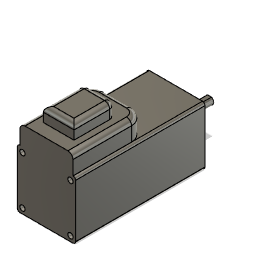
Assembly v15 (Autodesk Fusion 360 archive; units mm, degrees)
design "NEMA 23 Integrated Easy Servo Motor 130w"
Autodesk Fusion 360 part; units mm, degrees
sketch "Sketch1" plane through (0, 0, 0) normal (0, 0, 1) x (1, 0, 0)
  line L0 (0, 0) -> (57.15, 0)
  line L1 (57.15, 0) -> (57.15, 57.15)
  line L2 (57.15, 57.15) -> (0, 57.15)
  line L3 (0, 57.15) -> (0, 0)
  circle A0 centre (52.125, 52.125) radius 2.6
  line L4 (28.575, 0) -> (28.575, 57.15) construction
  line L5 (0, 28.575) -> (57.15, 28.575) construction
  circle A1 centre (5.025, 52.125) radius 2.6
  circle A2 centre (5.025, 5.025) radius 2.6
  circle A3 centre (52.125, 5.025) radius 2.6
  circle A4 centre (28.575, 28.575) radius 19.05
  line L6 (2.575, 57.15) -> (54.575, 57.15)
  line L7 (54.575, 57.15) -> (54.575, 76)
  line L8 (54.575, 76) -> (2.575, 76)
  line L9 (2.575, 76) -> (2.575, 57.15)
  circle A5 centre (28.575, 28.575) radius 4
  line L10 (26.6385, 32.075) -> (30.5115, 32.075)
  line L11 (13.575, 76) -> (43.575, 76)
  line L12 (43.575, 76) -> (43.575, 89.67)
  line L13 (43.575, 89.67) -> (13.575, 89.67)
  line L14 (13.575, 89.67) -> (13.575, 76)
  point P0 (47.5479, 45.3005)
  dimension "d1" = 57.15
  dimension "d2" = 57.15
  dimension "d3" = 5.2
  dimension "d5" = 5.2
  dimension "d6" = 47.1
  dimension "d8" = 5.2
  dimension "d10" = 47.1
  dimension "d12" = 5.2
  dimension "d13" = 47.1
  dimension "d14" = 47.1
  dimension "d15" = 38.1
  dimension "d16" = 76
  dimension "d17" = 8
  dimension "d19" = 3.5
  dimension "d20" = 52
  dimension "d21" = 13.67
  dimension "d22" = 30
  constraint horizontal L0
  constraint vertical L1
  constraint horizontal L2
  constraint vertical L3
  constraint coincident L0.start L3.end
  constraint midpoint L0 L4.start
  constraint midpoint L2 L4.end
  constraint midpoint L3 L5.start
  constraint midpoint L1 L5.end
  constraint symmetric A0 L4 A1
  constraint symmetric L5 A1.centre A2.centre
  constraint midpoint L5 A4.centre
  constraint horizontal L6
  constraint vertical L7
  constraint horizontal L8
  constraint vertical L9
  constraint coincident L2 L6.start
  constraint concentric A4 A5
  constraint coincident A5 L10.start
  constraint coincident A5 L10.end
  constraint perpendicular L4 L10
  constraint symmetric L4 L7 L9
  constraint horizontal L11
  constraint vertical L12
  constraint horizontal L13
  constraint vertical L14
  constraint coincident L8 L11.start
  constraint symmetric L4 L12 L14
  measures "d1" distance of L0.start L0.end
  measures "d2" distance of L0.start L2.end
  measures "d3" diameter of A0
  measures "d5" diameter of A1
  measures "d6" distance of A0.centre A1.centre
  measures "d8" diameter of A2
  measures "d10" distance of A1.centre A2.centre
  measures "d12" diameter of A3
  measures "d13" horizontal distance of A2.centre A3.centre
  measures "d14" distance of A0.centre A3.centre
  measures "d15" diameter of A4
  measures "d16" distance of L0 L8
  measures "d17" diameter of A5
  measures "d19" distance of L5 L10
  measures "d20" distance of L7.end L8.end
  measures "d21" distance of L11.start L13.end
  measures "d22" distance of L12.end L13.end
extrude "Extrude1" add sketch "Sketch1" along normal blind 127 contours L0 L1 L2 L3 L6 | A4 | A5 L10 | A5 L10
fillet "Fillet1" radius 2.5 4 edges at (57.15, 57.15, 63.5) (57.15, 0, 63.5) (0, 0, 63.5) (0, 57.15, 63.5)
extrude "Extrude2" add sketch "Sketch1" against normal blind 70 from surface at 127 contours L2 L6 L7 L8 L9 L11
fillet "Fillet2" radius 12.5 2 edges at (54.575, 66.575, 57) (2.575, 66.575, 57)
fillet "Fillet2" radius 5 3 edges at (54.575, 76, 92) (28.575, 76, 57) (2.575, 76, 92)
extrude "Extrude3" add sketch "Sketch1" along normal blind 40 from surface at 75 contours L8 L11 L12 L13 L14
fillet "Fillet3" radius 5 6 edges at (43.575, 89.67, 95) (43.575, 82.835, 75) (13.575, 82.835, 75) (28.575, 89.67, 75) (13.575, 89.67, 95) (28.575, 89.67, 115)
extrude "Extrude4" add sketch "Sketch1" against normal blind 2 contours A4 | A5 L10 | A5 L10
extrude "Extrude5" add sketch "Sketch1" against normal blind 33 contours A5 L10 picked at (29.5161, 29.5962)
extrude "Extrude6" add sketch "Sketch1" against normal blind 6 contours A5 L10 picked at (28.1041, 32.1557)
equation "d10 = d6"
equation "d12 = d3"
equation "d13 = d6"
equation "d14 = d6"
equation "d19 = 7.5 mm - ( d17 / 2 )"
equation "d44 = ( -1 * ( 33 - 27 ) ) * 1 mm"

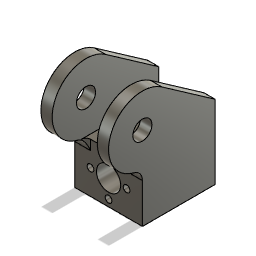
design "Lead Screw Nut Mount"
Autodesk Fusion 360 part; units mm, degrees
sketch "Sketch1" plane through (0, 0, 0) normal (0, 0, 1) x (1, 0, 0)
  circle A0 centre (0, 0) radius 5.375
  line L0 (0, 0) -> (0, 45)
  line L1 (0, 0) -> (55, 0)
  line L2 (-15, -11) -> (15, -11)
  line L3 (15, -11) -> (15, 11)
  line L4 (15, 11) -> (-15, 11)
  line L5 (-15, 11) -> (-15, -11)
  circle A1 centre (0, 8) radius 1.5
  circle A2 centre (-8, 0) radius 1.5
  circle A3 centre (0, -8) radius 1.5
  circle A4 centre (8, 0) radius 1.5
  dimension "d5" = 10.75
  dimension "d9" = 3
  dimension "d10" = 8
  dimension "d12" = 360
  dimension "d14" = 3
  dimension "d27" = 30
  constraint coincident A0.centre L0.start
  constraint vertical L0
  constraint perpendicular L0 L1
  constraint horizontal L2
  constraint vertical L3
  constraint horizontal L4
  constraint vertical L5
  constraint symmetric L0 L3 L5
  constraint symmetric L1 L2 L4
  constraint coincident L0 A1.centre
  measures "d5" diameter of A0
  measures "d9" diameter of A1
  measures "d10" distance of A0.centre A1.centre
  measures "d14" distance of L2 A3.centre
  measures "d27" distance of L3 L5
extrude "Extrude1" add sketch "Sketch1" along normal blind 32.25 contours A0 L0 L1 L2 L3 L4 L5 A1 A4 | A0 L0 L1 L3 L4 A1 A4
sketch "Sketch2" plane through (15, 0, 0) normal (1, 0, 0) x (0, 0, -1)
  line L0 (0, -11) -> (0, 11)
  line L1 (0, 11) -> (-32.25, 11)
  line L2 (-32.25, 11) -> (-32.25, -11)
  line L3 (-32.25, -11) -> (0, -11)
  circle A0 centre (-32.25, 26) radius 4.25
  circle A1 centre (-32.25, 26) radius 15
  line L4 (0, 11) -> (0, 21.7299)
  line L5 (0, 21.7299) -> (-23.6464, 38.2873)
  dimension "d20" = 8.5
  dimension "d21" = 15
  dimension "d28" = 30
  dimension "d34" = 125
  constraint concentric A0 A1
  constraint coincident L1.end A1
  constraint coincident L0.end L1.start
  constraint perpendicular L1 L4
  constraint coincident A1 L5.end
  constraint tangent A1 L5
  measures "d20" diameter of A0
  measures "d21" distance of L1 A0.centre
  measures "d28" diameter of A1
  measures "d34" angle of L4 L5
extrude "Extrude2" add sketch "Sketch2" against normal blind 5 contours L1 A1 L4 L5 | A1
ref_plane "WorkPlane1" through (0, 16.75, 24.9478) normal (1, 0, 0) x (0, 1, 0)
mirror "Mirror1" about plane through (0, 16.75, 24.9478) normal (1, 0, 0) of "Extrude2"
fillet "Fillet1" radius 5 2 edges at (-12.5, 11, 32.25) (12.5, 11, 32.25)
fillet "Fillet2" radius 2 1 edges at (-10, 8.8175, 32.25)
equation "Screw_Nut_Dia = 10 mm"
equation "Screw_Nut_bolt_Dia = 3 mm"
equation "Screw_Nut_Bolt_Pattern = 16 mm"
equation "d5 = Screw_Nut_Dia + 0.75 mm"
equation "d9 = Screw_Nut_bolt_Dia"
equation "d10 = Screw_Nut_Bolt_Pattern / 2"
equation "d13 = Screw_Nut_bolt_Dia"
equation "d14 = d13"
equation "d28 = 22 mm + 8 mm"
equation "d34 = 180 deg - 55 deg"

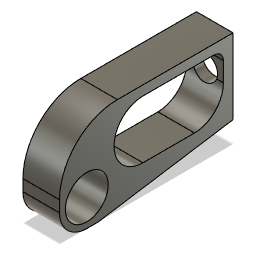
design "Connector 2"
Autodesk Fusion 360 part; units mm, degrees
sketch "Sketch1" plane through (0, 0, 0) normal (0, 1, 0) x (1, 0, 0)
  line L0 (0, 0) -> (19, 0)
  line L1 (19, 0) -> (19, 90)
  line L2 (19, 90) -> (0, 90)
  line L3 (0, 90) -> (0, 0)
  dimension "d1" = 19
  dimension "d2" = 90
  constraint horizontal L0
  constraint vertical L1
  constraint horizontal L2
  constraint vertical L3
  constraint coincident L0.start L3.end
  measures "d1" distance of L0.start L0.end
  measures "d2" distance of L0.start L2.end
extrude "Extrude1" add sketch "Sketch1" along normal blind 50
sketch "Sketch2" plane through (19, 0, 0) normal (1, 0, 0) x (0, 0, -1)
  line L0 (0, 0) -> (90, 0)
  line L1 (90, 0) -> (90, 50)
  line L2 (90, 50) -> (0, 50)
  line L3 (0, 50) -> (0, 0)
  circle A0 centre (14.125, 14.125) radius 11.125
  line L4 (28.25, 45) -> (85, 45)
  line L5 (85, 45) -> (85, 15)
  line L6 (85, 15) -> (28.25, 15)
  line L7 (28.25, 15) -> (28.25, 45)
  circle A1 centre (14.125, 14.125) radius 14.125
  dimension "d5" = 22.25
  dimension "d7" = 5
  dimension "d8" = 15
  dimension "d9" = 5
  dimension "d10" = 30
  dimension "d24" = 3
  constraint horizontal L4
  constraint vertical L5
  constraint horizontal L6
  constraint vertical L7
  constraint tangent L3 A1
  constraint tangent L0 A1
  constraint tangent L7 A1
  measures "d5" diameter of A0
  measures "d7" distance of L2 L4
  measures "d8" distance of L0 L6
  measures "d9" distance of L1 L5
  measures "d10" distance of L4 L6
extrude "Extrude2" cut sketch "Sketch2" against normal up to surface (19 mm away) contours L0 L3 A1 | A0 | L4 L5 L6 L7
fillet "Fillet1" radius 30 1 edges at (9.5, 50, 0)
sketch "Sketch3" plane through (0, 0, -90) normal (0, 0, -1) x (-1, 0, 0)
  line L0 (-19, 0) -> (0, 0)
  line L1 (0, 0) -> (0, 50)
  line L2 (0, 50) -> (-19, 50)
  line L3 (-19, 50) -> (-19, 0)
  circle A0 centre (-9.5, 32.5) radius 6.5
  line L4 (-9.5, 50) -> (-9.5, 0) construction
  line L5 (-19, 32.5) -> (0, 32.5) construction
  dimension "d17" = 13
  dimension "d29" = 17.5
  constraint midpoint L2 L4.start
  constraint midpoint L0 L4.end
  constraint coincident A0.centre L4
  constraint coincident A0.centre L5
  constraint horizontal L5
  constraint coincident L3 L5.start
  constraint coincident L1 L5.end
  measures "d17" diameter of A0
  measures "d29" distance of L2 L5
extrude "Extrude3" cut sketch "Sketch3" against normal up to surface (5 mm away) contours A0
fillet "Fillet2" radius 15 1 edges at (9.5, 15, -85)
fillet "Fillet2" radius 5 1 edges at (9.5, 45, -85)
fillet "Fillet3" radius 15 2 edges at (9.5, 45, -28.25) (9.5, 15, -28.25)
chamfer "Chamfer1" distance 11 distance2 70 1 edges at (9.5, 0, -90) measured on face at (9.6619, 8.6727, -90)
equation "d6 = d5"

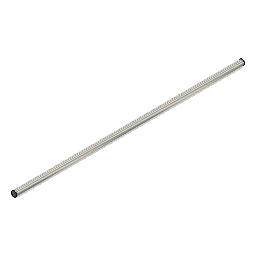
design "8mm T8 Lead Screw (345mm)"
Autodesk Fusion 360 part; units mm, degrees
sketch "Sketch1" plane through (0, 0, 0) normal (0, 0, 1) x (1, 0, 0)
  circle A0 centre (0, 0) radius 4
  dimension "d1" = 8
  constraint coincident A0.centre origin
  measures "d1" diameter of A0
extrude "Extrude1" add sketch "Sketch1" along normal blind 345
thread "Thread1" "ISO Metric Trapezoidal Threads 8.0 TR8x1.5 7e" major diameter 7.925 minor diameter 6.0605 pitch 1.5 angle 30 resizes the face on face at (-1.5959, -3.6679, 230)

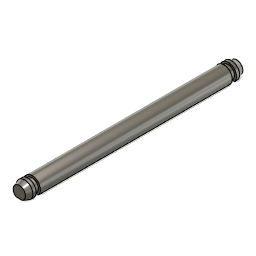
design "Pin Long (80mm)"
Autodesk Fusion 360 part; units mm, degrees
sketch "Sketch1" plane through (0, 0, 0) normal (0, 0, 1) x (1, 0, 0)
  line L0 (0, 0) -> (5.9867, 0)
  arc A0 (5.9867, 0) -> (0, 0) centre (2.9933, 2.5) ccw
  arc A1 (4.6516, 0) -> (1.335, 0) centre (2.9933, 2.5) ccw
  arc A2 (17.1516, 0) -> (13.835, 0) centre (15.4933, 2.5) ccw
  line L1 (12.5, 0) -> (18.4867, 0)
  arc A3 (18.4867, 0) -> (12.5, 0) centre (15.4933, 2.5) ccw
  arc A4 (29.6516, 0) -> (26.335, 0) centre (27.9933, 2.5) ccw
  line L2 (25, 0) -> (30.9867, 0)
  arc A5 (30.9867, 0) -> (25, 0) centre (27.9933, 2.5) ccw
  point P0 (12.5, 0)
  point P1 (25, 0)
  dimension "d1" = 3.9
  dimension "d2" = 2.5
  dimension "d13" = 6
  dimension "d16" = 25
  dimension "d17" = 0
  constraint coincident L0.start A0.end
  constraint horizontal L0
  constraint concentric A0 A1
  constraint coincident L0 A1.end
  constraint coincident L0 A1.start
  measures "d1" radius of A0
  measures "d2" distance of L0 A0.centre
  measures "d13" diameter of A1
extrude "Extrude1" add sketch "Sketch1" along normal blind 102 contours L0 A0 A1 | L0 A1 makes body 1
extrude "Extrude2" cut sketch "Sketch1" against normal blind 2 from surface at 6 contours L0 A0 A1 bodies 1
ref_plane "WorkPlane1" through (2.9933, 3.9289, 51) normal (0, 0, 1) x (1, 0, 0)
mirror "Mirror1" about plane through (2.9933, 3.9289, 51) normal (0, 0, 1) of "Extrude2"
extrude "Extrude3" add sketch "Sketch1" along normal blind 41 separate body contours A2 L1 | A2 L1 A3 makes body 2
extrude "Extrude4" cut sketch "Sketch1" against normal blind 2 from surface at 6 contours A2 L1 A3 bodies 2
ref_plane "WorkPlane2" through (15.4933, 3.9289, 20.5) normal (0, 0, 1) x (1, 0, 0)
mirror "Mirror2" about plane through (15.4933, 3.9289, 20.5) normal (0, 0, 1) of "Extrude4"
chamfer "Chamfer3" distance 2.5 distance2 1 1 edges at (15.4933, 6.4, 0) measured on face at (12.3817, 0.1488, 2.6667) on bodies 1 2
chamfer "Chamfer3" distance 2.5 distance2 1 1 edges at (2.9933, 6.4, 0) measured on face at (-0.1183, 0.1488, 2.6667) on bodies 1 2
chamfer "Chamfer3" distance 1 distance2 2.5 2 edges at (15.4933, 6.4, 41) (2.9933, 6.4, 102) measured on face at (16.772, 1.0681, 41) measured on face at (3.5688, 2.2017, 102) on bodies 1 2
hidden bodies 2
equation "d7 = Long_Pin + End_Thickness * 2"
equation "C_Clip_Thickness = 2 mm"
equation "End_Thickness = 4 mm + C_Clip_Thickness"
equation "Long_Pin = 90 mm"
equation "Short_Pin = 29 mm"
equation "d18 = End_Thickness"
equation "d19 = -C_Clip_Thickness"
equation "d25 = Short_Pin + End_Thickness * 2"
equation "d27 = End_Thickness"
equation "d28 = -C_Clip_Thickness"

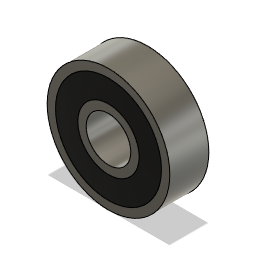
design "608 Bearings"
Autodesk Fusion 360 part; units mm, degrees
sketch "Sketch1" plane through (0, 0, 0) normal (0, 0, 1) x (1, 0, 0)
  circle A0 centre (0, 0) radius 11
  circle A1 centre (0, 0) radius 9.5
  circle A2 centre (0, 0) radius 4
  circle A3 centre (0, 0) radius 5.5
  dimension "d1" = 22
  dimension "d2" = -1.5
  dimension "d3" = 8
  dimension "d4" = 1.5
  constraint coincident A0.centre A1.centre
  measures "d1" diameter of A0
  measures "d3" diameter of A2
extrude "Extrude1" add sketch "Sketch1" along normal blind 7 makes body 1 at (5.4727, -0.5476, 4.6667) makes body 2 at (10.9453, -1.0952, 4.6667)
extrude "Extrude2" add sketch "Sketch1" along normal blind 7 separate body contours A1 makes body 3

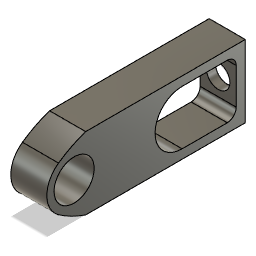
design "Connectors"
Autodesk Fusion 360 part; units mm, degrees
sketch "Sketch1" plane through (0, 0, 0) normal (0, 1, 0) x (1, 0, 0)
  line L0 (0, 0) -> (20, 0)
  line L1 (20, 0) -> (20, 110)
  line L2 (20, 110) -> (0, 110)
  line L3 (0, 110) -> (0, 0)
  dimension "d1" = 20
  dimension "d2" = 110
  constraint horizontal L0
  constraint vertical L1
  constraint horizontal L2
  constraint vertical L3
  constraint coincident L0.start L3.end
  measures "d1" distance of L0.start L0.end
  measures "d2" distance of L0.start L2.end
extrude "Extrude1" add sketch "Sketch1" along normal blind 40
sketch "Sketch2" plane through (20, 0, 0) normal (1, 0, 0) x (0, 0, -1)
  line L0 (0, 0) -> (110, 0)
  line L1 (110, 0) -> (110, 40)
  line L2 (110, 40) -> (0, 40)
  line L3 (0, 40) -> (0, 0)
  circle A0 centre (15.125, 20) radius 11.125
  line L4 (60, 35) -> (105, 35)
  line L5 (105, 35) -> (105, 5)
  line L6 (105, 5) -> (60, 5)
  line L7 (60, 5) -> (60, 35)
  line L8 (0, 20) -> (13, 20) construction
  circle A1 centre (15.125, 20) radius 15.125
  arc A2 (60, 40) -> (6.4846, 32.414) centre (40.7607, -16.8318) ccw
  arc A3 (6.4846, 7.586) -> (60, 0) centre (40.7607, 56.8318) ccw
  dimension "d5" = 22.25
  dimension "d7" = 5
  dimension "d8" = 5
  dimension "d9" = 5
  dimension "d10" = 30
  dimension "d11" = 45
  dimension "d24" = 4
  dimension "d25" = 60
  constraint horizontal L4
  constraint vertical L5
  constraint horizontal L6
  constraint vertical L7
  constraint midpoint L3 L8.start
  constraint perpendicular L3 L8
  constraint coincident A0.centre L8
  constraint tangent A1 A2
  constraint coincident A1 A2.end
  constraint coincident L2 A2.start
  constraint coincident L7 A2.start
  constraint symmetric L8 A2.start A3.end
  constraint symmetric L8 A2.end A3.start
  constraint symmetric L8 A2 A3
  constraint tangent L3 A1
  measures "d5" diameter of A0
  measures "d7" distance of L2 L4
  measures "d8" distance of L0 L6
  measures "d9" distance of L1 L5
  measures "d10" distance of L4 L6
  measures "d11" distance of L5 L7
  measures "d25" radius of A2
extrude "Extrude2" cut sketch "Sketch2" against normal up to surface (20 mm away) contours L0 L3 A1 A3 | L2 L3 A1 A2 | A0 | L4 L5 L6 L7
sketch "Sketch3" plane through (0, 0, -110) normal (0, 0, -1) x (-1, 0, 0)
  line L0 (-20, 0) -> (0, 0)
  line L1 (0, 0) -> (0, 40)
  line L2 (0, 40) -> (-20, 40)
  line L3 (-20, 40) -> (-20, 0)
  circle A0 centre (-10, 20) radius 6.5
  line L4 (-10, 40) -> (-10, 0) construction
  line L5 (-20, 20) -> (0, 20) construction
  dimension "d17" = 13
  constraint midpoint L2 L4.start
  constraint midpoint L0 L4.end
  constraint midpoint L3 L5.start
  constraint midpoint L1 L5.end
  constraint coincident A0.centre L4
  constraint coincident A0.centre L5
  measures "d17" diameter of A0
extrude "Extrude3" cut sketch "Sketch3" against normal up to surface (5 mm away) contours A0
fillet "Fillet2" radius 5 2 edges at (10, 35, -105) (10, 5, -105)
fillet "Fillet3" radius 15 2 edges at (10, 35, -60) (10, 5, -60)

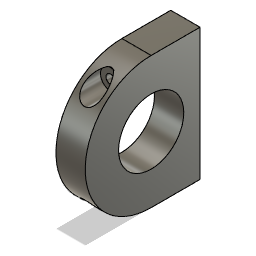
design "Pedal Mounting Ears"
Autodesk Fusion 360 part; units mm, degrees
sketch "Sketch1" plane through (0, 0, 0) normal (1, 0, 0) x (0, 0, -1)
  line L0 (-16.6875, 45) -> (0, 45)
  line L1 (0, 45) -> (0, 0)
  line L2 (0, 0) -> (-16.6875, 0)
  arc A0 (-16.6875, 45) -> (-16.6875, 0) centre (-16.6875, 22.5) ccw
  circle A1 centre (-16.6875, 22.5) radius 11.125
  line L3 (0, 22.5) -> (-29, 22.5) construction
  circle A2 centre (-16.6875, 22.5) radius 9.125
  dimension "d1" = 22.25
  dimension "d2" = 45
  dimension "d3" = 16.6875
  dimension "d4" = -2
  constraint horizontal L0
  constraint coincident L1.end L2.start
  constraint perpendicular L0 L1
  constraint perpendicular L1 L2
  constraint tangent L2 A0
  constraint tangent L0 A0
  constraint midpoint L1 L3.start
  constraint perpendicular L1 L3
  constraint coincident A0.centre L3
  constraint coincident A0.centre A1.centre
  measures "d1" diameter of A1
  measures "d2" distance of L0 L2
  measures "d3" distance of L1 A0.centre
extrude "Extrude2" add sketch "Sketch1" along normal blind 10 contours L0 L1 L2 A0
sketch "Sketch2" plane through (0, 0, 0) normal (0, 0, -1) x (-1, 0, 0)
  line L0 (0, 45) -> (-10, 45)
  line L1 (-10, 0) -> (0, 0)
  circle A0 centre (-5, 5.2) radius 3.5
  line L2 (-5, 0) -> (-5, 4) construction
  circle A1 centre (-5, 5.2) radius 1.6
  line L3 (0, 0) -> (0, 45)
  line L4 (-10, 45) -> (-10, 0)
  dimension "d13" = 7
  dimension "d14" = 5.2
  dimension "d17" = 3.2
  constraint midpoint L1 L2.start
  constraint perpendicular L1 L2
  constraint coincident A0.centre L2
  constraint concentric A0 A1
  measures "d13" diameter of A0
  measures "d14" distance of L1 A0.centre
  measures "d17" diameter of A1
extrude "Extrude4" cut sketch "Sketch2" against normal blind 40 contours A0 | A1
extrude "Extrude5" add sketch "Sketch2" against normal blind 25.5 contours A0
ref_plane "WorkPlane1" through (5, 22.5, 8.3438) normal (0, -1, 0) x (0, 0, -1)
mirror "Mirror1" about plane through (5, 22.5, 8.3438) normal (0, -1, 0) of "Extrude4", "Extrude5"
equation "d3 = d1 * 0.75"
equation "d14 = d13 / 2 + 1.7 mm"

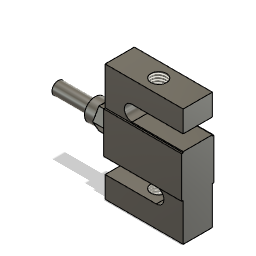
design "Load Cell (300 kg)"
Autodesk Fusion 360 part; units mm, degrees
sketch "Sketch1" plane through (0, 0, 0) normal (0, 0, 1) x (1, 0, 0)
  line L0 (0, 0) -> (50.75, 0)
  line L1 (50.75, 0) -> (50.75, 52.25)
  line L2 (50.75, 52.25) -> (12.5, 52.25)
  line L3 (12.5, 52.25) -> (12.5, 62.25)
  line L4 (12.5, 62.25) -> (50.75, 62.25)
  line L5 (50.75, 62.25) -> (50.75, 76.25)
  line L6 (50.75, 76.25) -> (0, 76.25)
  line L7 (0, 76.25) -> (0, 24)
  line L8 (0, 24) -> (38.25, 24)
  line L9 (38.25, 24) -> (38.25, 14)
  line L10 (38.25, 14) -> (0, 14)
  line L11 (0, 14) -> (0, 0)
  line L12 (0, 24.75) -> (50.75, 24.75)
  line L13 (50.75, 51.5) -> (0, 51.5)
  dimension "d1" = 76.25
  dimension "d2" = 14
  dimension "d3" = 10
  dimension "d4" = 50.75
  dimension "d5" = 12.5
  dimension "d6" = 0.75
  dimension "d7" = 0.75
  constraint coincident L0.start L11.end
  constraint horizontal L0
  constraint perpendicular L0 L1
  constraint perpendicular L1 L2
  constraint perpendicular L2 L3
  constraint perpendicular L3 L4
  constraint perpendicular L4 L5
  constraint perpendicular L5 L6
  constraint perpendicular L6 L7
  constraint perpendicular L7 L8
  constraint perpendicular L8 L9
  constraint perpendicular L9 L10
  constraint perpendicular L0 L11
  constraint equal L5 L11
  constraint equal L3 L9
  constraint collinear L7 L11
  constraint collinear L1 L5
  constraint equal L2 L10
  constraint coincident L7 L12.start
  constraint coincident L1 L12.end
  constraint perpendicular L1 L12
  constraint coincident L1 L13.start
  constraint coincident L7 L13.end
  constraint perpendicular L7 L13
  measures "d1" distance of L0 L6
  measures "d2" distance of L4.end L5.end
  measures "d3" distance of L2.end L3.end
  measures "d4" distance of L5.end L6.end
  measures "d5" distance of L1 L9
  measures "d6" distance of L8 L12
  measures "d7" distance of L2 L13
extrude "Extrude1" add sketch "Sketch1" along normal mid plane 19
extrude "Extrude2" add sketch "Sketch1" along normal mid plane 21 contours L1 L7 L12 L13
sketch "Sketch2" plane through (0, 0, 0) normal (-1, 0, 0) x (0, 0, 1)
  line L0 (9.5, 51.5) -> (9.5, 76.25)
  line L1 (9.5, 76.25) -> (-9.5, 76.25)
  line L2 (-9.5, 76.25) -> (-9.5, 51.5)
  line L3 (-9.5, 51.5) -> (-10.5, 51.5)
  line L4 (-10.5, 51.5) -> (-10.5, 24.75)
  line L5 (-10.5, 24.75) -> (-9.5, 24.75)
  line L6 (-9.5, 24.75) -> (-9.5, 24)
  line L7 (-9.5, 24) -> (9.5, 24)
  line L8 (9.5, 24) -> (9.5, 24.75)
  line L9 (9.5, 24.75) -> (10.5, 24.75)
  line L10 (10.5, 24.75) -> (10.5, 51.5)
  line L11 (10.5, 51.5) -> (9.5, 51.5)
  line L12 (8.0829, 38.125) -> (4.0415, 45.125)
  line L13 (4.0415, 45.125) -> (-4.0415, 45.125)
  line L14 (-4.0415, 45.125) -> (-8.0829, 38.125)
  line L15 (-8.0829, 38.125) -> (-4.0415, 31.125)
  line L16 (-4.0415, 31.125) -> (4.0415, 31.125)
  line L17 (4.0415, 31.125) -> (8.0829, 38.125)
  line L18 (-9.5, 0) -> (9.5, 0)
  line L19 (0, 76.25) -> (0, 24)
  circle A0 centre (0, 38.125) radius 4.1
  circle A1 centre (0, 38.125) radius 7
  point P0 (0, 38.125)
  dimension "d12" = 7
  dimension "d13" = 38.125
  dimension "d14" = 8.2
  dimension "d15" = 14
  constraint horizontal L16
  constraint coincident P0 L19
  constraint coincident P0 A0.centre
  constraint concentric A0 A1
  measures "d12" distance of P0 L17
  measures "d13" distance of P0 L18
  measures "d14" diameter of A0
  measures "d15" diameter of A1
extrude "Extrude3" add sketch "Sketch2" along normal blind 9.5 contours L13 L14 A1 | L19 A0 A1 | L12 L13 A1 | L19 A0 A1 | L19 A0 | L19 A0 | L12 L17 A1 | L14 L15 A1 | L15 L16 A1 | L16 L17 A1
extrude "Extrude4" add sketch "Sketch2" along normal blind 16 contours L19 A0 A1 | L19 A0 A1 | L19 A0 | L19 A0
extrude "Extrude5" add sketch "Sketch2" along normal blind 40 contours L19 A0 | L19 A0
fillet "Fillet1" radius 5 4 edges at (38.25, 14, 0) (38.25, 24, 0) (12.5, 62.25, 0) (12.5, 52.25, 0)
sketch "Sketch3" plane through (0, 76.25, 0) normal (0, 1, 0) x (-1, 0, 0)
  line L0 (0, -9.5) -> (0, 9.5)
  line L1 (0, 9.5) -> (-50.75, 9.5)
  line L2 (-50.75, 9.5) -> (-50.75, -9.5)
  line L3 (-50.75, -9.5) -> (0, -9.5)
  circle A0 centre (-25.375, 0) radius 6
  line L4 (0, 4.0415) -> (0, -4.0415)
  line L5 (-50.75, 0) -> (0, 0)
  dimension "d24" = 25.375
  dimension "d25" = 12
  constraint coincident A0.centre L5
  measures "d24" distance of A0.centre L4
  measures "d25" diameter of A0
extrude "Extrude6" cut sketch "Sketch3" against normal up to surface (14 mm away) contours A0 L5 | A0 L5
extrude "Extrude7" cut sketch "Sketch3" along normal up to surface (14 mm away) from surface at -76.25 contours A0 L5 | A0 L5
thread "Thread1" "ISO Metric profile 12.0 M12x1.75 6H" major diameter 12.2265 minor diameter 10.2735 pitch 1.75 angle 60 resizes the face on face at (19.3825, 66.9167, -0.2991)
thread "Thread2" "ISO Metric profile 12.0 M12x1.75 6H" major diameter 12.2265 minor diameter 10.2735 pitch 1.75 angle 60 resizes the face on face at (19.4048, 4.6667, -0.5974)
equation "d8 = ( 19 / 2 ) * 1 mm"
equation "d10 = ( 21 / 2 ) * 1 mm"
equation "d12 = ( 14 / 2 ) * 1 mm"
equation "d13 = d1 / 2"
equation "d24 = d4 / 2"

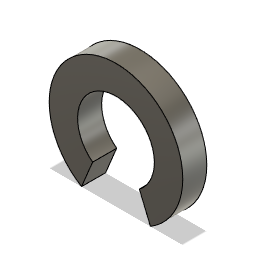
design "C Clip"
Autodesk Fusion 360 part; units mm, degrees
sketch "Sketch1" plane through (0, 0, 0) normal (0, 0, 1) x (1, 0, 0)
  line L0 (-1.75, -2.281) -> (-2.5794, -4.2833)
  line L1 (1.75, -2.281) -> (2.5794, -4.2833)
  line L2 (0, 0) -> (0, -5) construction
  arc A0 (2.5794, -4.2833) -> (-2.5794, -4.2833) centre (0, 0) ccw
  arc A1 (1.75, -2.281) -> (-1.75, -2.281) centre (0, 0) ccw
  dimension "d7" = 5.75
  dimension "d8" = 10
  dimension "d9" = 45
  dimension "d10" = 3.5
  constraint coincident L2.start A0.centre
  constraint concentric A0 A1
  constraint vertical L2
  constraint symmetric L0 L1 L2
  measures "d7" diameter of A1
  measures "d8" diameter of A0
  measures "d9" angle of L0 L1
  measures "d10" distance of L1.start L0.start
extrude "Extrude1" add sketch "Sketch1" along normal blind 1.8

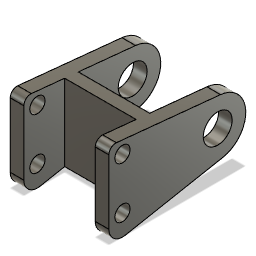
design "Pedal Connector"
Autodesk Fusion 360 part; units mm, degrees
sketch "Sketch3" plane through (0, 0, 0) normal (1, 0, 0) x (0, 0, -1)
  circle A0 centre (4, 22) radius 2.25
  circle A1 centre (4, 7) radius 2.25
  line L0 (0, 0) -> (0, 26)
  circle A2 centre (32, 14.5) radius 4.25
  line L1 (12, 24.7968) -> (12, 2.288)
  line L2 (4, 22) -> (4, 7) construction
  line L3 (4, 14.5) -> (32, 14.5) construction
  circle A3 centre (32, 14.5) radius 8.25
  line L4 (0, 26) -> (32.8231, 22.7088)
  line L5 (0, 0) -> (33.5452, 6.396)
  line L6 (16, 24.3957) -> (16, 0.2355)
  dimension "d16" = 4.5
  dimension "d17" = 4.5
  dimension "d18" = 8.5
  dimension "d21" = 4
  dimension "d22" = 4
  dimension "d23" = 15
  dimension "d25" = 4
  dimension "d28" = 8
  dimension "d29" = 7
  dimension "d30" = 90
  dimension "d32" = 4
  dimension "d43" = 4
  dimension "d44" = 16
  constraint coincident L0.start L5.start
  constraint vertical L0
  constraint coincident A0.centre L2.start
  constraint coincident A1.centre L2.end
  constraint midpoint L2 L3.start
  constraint coincident A2.centre L3.end
  constraint parallel L0 L1
  constraint coincident A3 L4.end
  constraint tangent A3 L4
  constraint coincident A3 L5.end
  constraint tangent A3 L5
  constraint coincident L1.start L4
  constraint coincident L1.end L5
  constraint coincident L4 L6.start
  constraint vertical L6
  measures "d16" diameter of A0
  measures "d17" diameter of A1
  measures "d18" diameter of A2
  measures "d21" distance of A1.centre L0
  measures "d22" distance of A0.centre L0
  measures "d23" distance of A0.centre A1.centre
  measures "d25" vertical distance of A0.centre L0.end
  measures "d28" distance of A0.centre L1
  measures "d29" vertical distance of L0.start A1.centre
  measures "d30" angle of L2 L3
  measures "d43" distance of L1 L6
  measures "d44" distance of A2.centre L6
extrude "Extrude2" add sketch "Sketch3" along normal blind 29
fillet "Fillet1" radius 4 1 edges at (14.5, 0, 0)
fillet "Fillet1" radius 2 1 edges at (14.5, 26, 0)
extrude "Extrude3" cut sketch "Sketch3" along normal blind 21 from surface at 4 contours L0 L1 L4 L5 | A3 L4 L5 L6 | A3
equation "d19 = d18 / 2 + 4 mm"
equation "d34 = 21 mm + ( 4 * 2 ) * 1 mm"
equation "d44 = ( 22 / 2 ) * 1 mm + 5 mm"

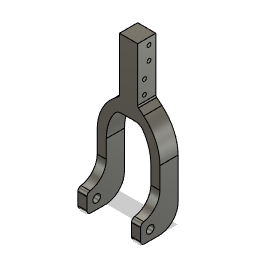
design "Pedal"
Autodesk Fusion 360 part; units mm, degrees
sketch "Pedal Shape" plane through (0, 0, 0) normal (0, 0, 1) x (1, 0, 0)
  line L0 (0, 0) -> (0, 89.4421)
  line L1 (0, 89.4421) -> (24.5, 110)
  line L2 (24.5, 110) -> (24.5, 170)
  line L3 (24.5, 170) -> (44.5, 170)
  line L4 (44.5, 170) -> (44.5, 110)
  line L5 (44.5, 110) -> (69, 89.4421)
  line L6 (69, 89.4421) -> (69, 0)
  line L7 (69, 0) -> (59, 0)
  line L8 (59, 0) -> (59, 84.779)
  line L9 (59, 84.779) -> (47.0825, 94.779)
  line L10 (47.0825, 94.779) -> (21.9175, 94.779)
  line L11 (21.9175, 94.779) -> (10, 84.779)
  line L12 (10, 84.779) -> (10, 0)
  line L13 (10, 0) -> (0, 0)
  dimension "d2" = 20
  dimension "d4" = 10
  dimension "d6" = 170
  dimension "d7" = 10
  dimension "d45" = 10
  dimension "d47" = 110
  dimension "d48" = 69
  constraint parallel L0 L2
  constraint perpendicular L2 L3
  constraint perpendicular L3 L4
  constraint perpendicular L3 L6
  constraint perpendicular L6 L7
  constraint perpendicular L7 L8
  constraint parallel L5 L9
  constraint perpendicular L8 L10
  constraint perpendicular L10 L12
  constraint coincident L0.start L13.end
  constraint equal L7 L13
  constraint equal L9 L11
  constraint equal L8 L12
  constraint equal L1 L5
  constraint equal L2 L4
  constraint horizontal L13
  constraint horizontal L7
  constraint collinear L7 L13
  constraint parallel L1 L11
  measures "d2" distance of L2.end L3.end
  measures "d4" distance of L0 L12
  measures "d6" distance of L3 L13
  measures "d7" distance of L5 L9
  measures "d45" distance of L10 L11.end
  measures "d47" distance of L1.end L13
  measures "d48" distance of L0 L6
extrude "Extrude1" add sketch "Pedal Shape" along normal blind 20
sketch "Pivot Point" plane through (0, 0, 0) normal (-1, 0, 0) x (0, 0, 1)
  line L0 (0, 89.4421) -> (0, 0)
  line L1 (0, 0) -> (20, 0)
  line L2 (20, 0) -> (20, 89.4421)
  line L3 (20, 89.4421) -> (0, 89.4421)
  circle A0 centre (30.625, 10.625) radius 4.25
  line L4 (20, 21.25) -> (41.25, 21.25)
  line L5 (41.25, 21.25) -> (41.25, 0)
  line L6 (41.25, 0) -> (20, 0)
  line L7 (20, 21.25) -> (20, 0)
  line L8 (30.625, 21.25) -> (30.625, 0) construction
  dimension "d12" = 8.5
  dimension "d13" = 10.625
  dimension "d16" = 21.25
  dimension "d17" = 21.25
  constraint coincident L2 L4.start
  constraint perpendicular L2 L4
  constraint perpendicular L4 L5
  constraint coincident L1.end L2.start
  constraint perpendicular L2 L6
  constraint midpoint L4 L8.start
  constraint midpoint L6 L8.end
  constraint coincident A0.centre L8
  measures "d12" diameter of A0
  measures "d13" distance of L1 A0.centre
  measures "d16" distance of L4.end L5.end
  measures "d17" distance of L5 L7
extrude "Extrude3" add sketch "Pivot Point" against normal blind 10 contours L2 L4 L5 L6 L7
fillet "Fillet1" radius 21.25 1 edges at (5, 21.25, 20)
fillet "Fillet1" radius 21.25 1 edges at (5, 0, 0)
ref_plane "WorkPlane1" through (34.5, 44.721, 10) normal (1, 0, 0) x (0, 1, 0)
mirror "Mirror1" about plane through (34.5, 44.721, 10) normal (1, 0, 0) of "Extrude3", "Fillet1"
sketch "Pedal and Connector Holes" plane through (44.5, 0, 0) normal (1, 0, 0) x (0, 0, -1)
  line L0 (0, 110) -> (0, 170)
  line L1 (0, 170) -> (-20, 170)
  line L2 (-20, 170) -> (-20, 110)
  line L3 (-20, 110) -> (0, 110)
  circle A0 centre (-12.5, 117.5) radius 2.125
  circle A1 centre (-12.5, 132.5) radius 2.125
  line L4 (-12.5, 105) -> (-12.5, 132.5) construction
  circle A2 centre (-7.5, 162.5) radius 2.125
  circle A3 centre (-7.5, 147.5) radius 2.125
  line L5 (-7.5, 162.5) -> (-7.5, 147.5) construction
  dimension "d27" = 4.25
  dimension "d28" = 4.25
  dimension "d29" = 15
  dimension "d30" = 7.5
  dimension "d33" = 7.5
  dimension "d34" = 4.25
  dimension "d35" = 4.25
  dimension "d36" = 15
  dimension "d37" = 7.5
  dimension "d38" = 7.5
  constraint coincident A1.centre L4.end
  constraint coincident A0.centre L4
  constraint vertical L4
  constraint coincident A2.centre L5.start
  constraint coincident A3.centre L5.end
  constraint vertical L5
  measures "d27" diameter of A0
  measures "d28" diameter of A1
  measures "d29" distance of A0.centre A1.centre
  measures "d30" distance of L3 A0.centre
  measures "d33" distance of L2 L4
  measures "d34" diameter of A3
  measures "d35" diameter of A2
  measures "d36" distance of A2.centre A3.centre
  measures "d37" distance of L0 A2.centre
  measures "d38" distance of L1 A2.centre
extrude "Extrude4" cut sketch "Pedal and Connector Holes" against normal up to surface (20 mm away) contours A0 | A1 | A2 | A3
fillet "Fillet2" radius 50 4 edges at (59, 84.779, 10) (10, 84.779, 10) (0, 89.4421, 10) (69, 89.4421, 10)
fillet "Fillet3" radius 10 2 edges at (47.0825, 94.779, 10) (21.9175, 94.779, 10)
fillet "Fillet4" radius 2.5 2 edges at (24.5, 110, 10) (44.5, 110, 10)
fillet "Fillet5" radius 4 4 edges at (64, 21.25, 41.25) (64, 0, 41.25) (5, 0, 41.25) (5, 21.25, 41.25)
equation "d13 = d12 * 1.25"
equation "d16 = d12 * 2.5"
equation "d17 = d16"
equation "d21 = d17"
equation "d23 = d17"
equation "d26 = -d4"
equation "d36 = d29"
equation "d37 = d33"
equation "d38 = d30"

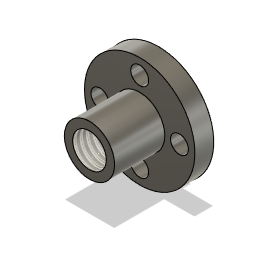
design "8mm Lead Screw Nut"
Autodesk Fusion 360 part; units mm, degrees
sketch "Sketch2" plane through (0, 0, 0) normal (0, 0, 1) x (1, 0, 0)
  circle A0 centre (0, 0) radius 5.05
  circle A1 centre (0, 0) radius 11.1
  line L0 (-35, 0) -> (41.5964, 0) construction
  line L1 (0, 35) -> (0, -35) construction
  circle A2 centre (0, 8) radius 1.8
  circle A3 centre (8, 0) radius 1.8
  circle A4 centre (0, -8) radius 1.8
  circle A5 centre (-8, 0) radius 1.8
  circle A6 centre (0, 0) radius 8 construction
  circle A7 centre (0, 0) radius 4
  dimension "d1" = 10.1
  dimension "d2" = 22.2
  dimension "d3" = 3.6
  dimension "d4" = 3.6
  dimension "d5" = 3.6
  dimension "d6" = 3.6
  dimension "d7" = 16
  dimension "d13" = 8
  constraint coincident A0.centre A1.centre
  constraint horizontal L0
  constraint vertical L1
  constraint coincident L1 A2.centre
  constraint coincident L0 A3.centre
  constraint coincident L1 A4.centre
  constraint coincident L0 A5.centre
  constraint coincident A2.centre A6
  constraint coincident A3.centre A6
  constraint coincident A4.centre A6
  constraint coincident A5.centre A6
  measures "d1" diameter of A0
  measures "d2" diameter of A1
  measures "d3" diameter of A2
  measures "d4" diameter of A3
  measures "d5" diameter of A4
  measures "d6" diameter of A5
  measures "d7" diameter of A6
  measures "d13" diameter of A7
extrude "Extrude1" add sketch "Sketch2" along normal blind 15.5 contours A0 | A7
extrude "Extrude2" add sketch "Sketch2" along normal blind 3.8 from surface at 1.6 contours A1
extrude "Extrude3" cut sketch "Sketch2" along normal up to surface (15.5 mm away) contours A7
thread "Thread1" "ISO Metric profile 8.0 M8x1.25 6H" major diameter 8.17 minor diameter 6.7795 pitch 1.25 angle 60 resizes the face on face at (3.995, -0.1994, 10.3333)

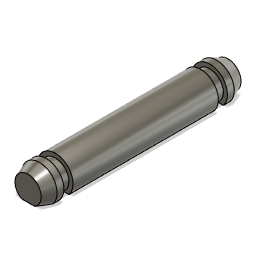
design "Pins Shrt (30mm)"
Autodesk Fusion 360 part; units mm, degrees
sketch "Sketch1" plane through (0, 0, 0) normal (0, 0, 1) x (1, 0, 0)
  line L0 (0, 0) -> (5.9867, 0)
  arc A0 (5.9867, 0) -> (0, 0) centre (2.9933, 2.5) ccw
  arc A1 (4.6516, 0) -> (1.335, 0) centre (2.9933, 2.5) ccw
  arc A2 (17.1516, 0) -> (13.835, 0) centre (15.4933, 2.5) ccw
  line L1 (12.5, 0) -> (18.4867, 0)
  arc A3 (18.4867, 0) -> (12.5, 0) centre (15.4933, 2.5) ccw
  arc A4 (29.6516, 0) -> (26.335, 0) centre (27.9933, 2.5) ccw
  line L2 (25, 0) -> (30.9867, 0)
  arc A5 (30.9867, 0) -> (25, 0) centre (27.9933, 2.5) ccw
  point P0 (12.5, 0)
  point P1 (25, 0)
  dimension "d1" = 3.9
  dimension "d2" = 2.5
  dimension "d13" = 6
  dimension "d16" = 25
  dimension "d17" = 0
  constraint coincident L0.start A0.end
  constraint horizontal L0
  constraint concentric A0 A1
  constraint coincident L0 A1.end
  constraint coincident L0 A1.start
  measures "d1" radius of A0
  measures "d2" distance of L0 A0.centre
  measures "d13" diameter of A1
extrude "Extrude1" add sketch "Sketch1" along normal blind 102 contours L0 A0 A1 | L0 A1 makes body 1
extrude "Extrude2" cut sketch "Sketch1" against normal blind 2 from surface at 6 contours L0 A0 A1 bodies 1
ref_plane "WorkPlane1" through (2.9933, 3.9289, 51) normal (0, 0, 1) x (1, 0, 0)
mirror "Mirror1" about plane through (2.9933, 3.9289, 51) normal (0, 0, 1) of "Extrude2"
extrude "Extrude3" add sketch "Sketch1" along normal blind 44 separate body contours A2 L1 | A2 L1 A3 makes body 2
extrude "Extrude4" cut sketch "Sketch1" against normal blind 2 from surface at 6 contours A2 L1 A3 bodies 2
ref_plane "WorkPlane2" through (15.4933, 3.9289, 22) normal (0, 0, 1) x (1, 0, 0)
mirror "Mirror2" about plane through (15.4933, 3.9289, 22) normal (0, 0, 1) of "Extrude4"
chamfer "Chamfer3" distance 2.5 distance2 1 1 edges at (15.4933, 6.4, 0) measured on face at (12.3817, 0.1488, 2.6667) on bodies 1 2
chamfer "Chamfer3" distance 2.5 distance2 1 1 edges at (2.9933, 6.4, 0) measured on face at (-0.1183, 0.1488, 2.6667) on bodies 1 2
chamfer "Chamfer3" distance 1 distance2 2.5 2 edges at (15.4933, 6.4, 44) (2.9933, 6.4, 102) measured on face at (16.772, 1.0681, 44) measured on face at (3.5688, 2.2017, 102) on bodies 1 2
hidden bodies 1
equation "d7 = Long_Pin + End_Thickness * 2"
equation "C_Clip_Thickness = 2 mm"
equation "End_Thickness = 4 mm + C_Clip_Thickness"
equation "Long_Pin = 90 mm"
equation "Short_Pin = 32 mm"
equation "d18 = End_Thickness"
equation "d19 = -C_Clip_Thickness"
equation "d25 = Short_Pin + End_Thickness * 2"
equation "d27 = End_Thickness"
equation "d28 = -C_Clip_Thickness"
